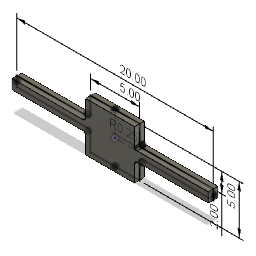
Table_17p1_Problem_5 (Autodesk Fusion 360 design; units mm, degrees)
Autodesk Fusion 360 part; units mm, degrees
sketch "Sketch1" plane through (0, 0, 0) normal (0, 0, 1) x (1, 0, 0)
  line L0 (0, 25) -> (25, 25)
  line L1 (25, 25) -> (25, 7.5)
  arc A0 (25, 7.5) -> (27.5, 5) centre (27.5, 7.5) ccw
  line L2 (27.5, 5) -> (100, 5)
  line L3 (100, 5) -> (100, 0)
  line L4 (0, 0) -> (0, 25) construction
  line L5 (0, 0) -> (100, 0) construction
  line L6 (0, -25) -> (25, -25)
  line L7 (25, -25) -> (25, -7.5)
  arc A1 (27.5, -5) -> (25, -7.5) centre (27.5, -7.5) ccw
  line L8 (27.5, -5) -> (100, -5)
  line L9 (100, -5) -> (100, 0)
  line L10 (0, 25) -> (-25, 25)
  line L11 (-25, 25) -> (-25, 7.5)
  arc A2 (-27.5, 5) -> (-25, 7.5) centre (-27.5, 7.5) ccw
  line L12 (-27.5, 5) -> (-100, 5)
  line L13 (-25, -25) -> (-25, -7.5)
  line L14 (-27.5, -5) -> (-100, -5)
  arc A3 (-25, -7.5) -> (-27.5, -5) centre (-27.5, -7.5) ccw
  line L15 (0, -25) -> (-25, -25)
  line L16 (-100, 5) -> (-100, 0)
  line L17 (-100, -5) -> (-100, 0)
  dimension "Fillet_Radius" = 2.5
  dimension "Shoulder_Height" = 20
  dimension "Shoulder_Width" = 50
  dimension "Total_Width" = 200
  dimension "Total_Height" = 50
  constraint horizontal L0
  constraint perpendicular L0 L1
  constraint tangent L1 A0
  constraint parallel L0 L2
  constraint vertical L3
  constraint tangent A0 L2
  constraint coincident L4.start L5.start
  constraint perpendicular L2 L4
  constraint perpendicular L3 L5
  constraint symmetric L0.start L5 L6.start
  constraint symmetric L0.end L5 L6.end
  constraint symmetric L1.end L5 L7.end
  constraint symmetric A0.end L5 A1.start
  constraint symmetric A0 L5 A1
  constraint symmetric L2.end L5 L8.end
  constraint symmetric L3.end L5 L9.end
  constraint symmetric L0.start L4 L10.start
  constraint symmetric L0.end L4 L10.end
  constraint symmetric L1.end L4 L11.end
  constraint symmetric A0.end L4 A2.start
  constraint symmetric A0 L4 A2
  constraint symmetric L2.end L4 L12.end
  constraint symmetric L3.end L4 L16.end
  constraint symmetric L4 L6.start L15.start
  constraint symmetric L4 L6.end L13.start
  constraint symmetric L4 L7.end L13.end
  constraint symmetric L4 A1.start L14.start
  constraint symmetric L4 A1 A3
  constraint symmetric L4 L8.end L14.end
  constraint symmetric L4 L3.end L16.end
  measures "Fillet_Radius" radius of A0
  measures "Shoulder_Height" distance of L0 L2
  measures "Shoulder_Width" distance of L1 L11
  measures "Total_Width" distance of L3 L16
  measures "Total_Height" distance of L0 L6
extrude "Extrude1" add sketch "Sketch1" along normal mid plane 10
equation "Thickness = 1 cm"
